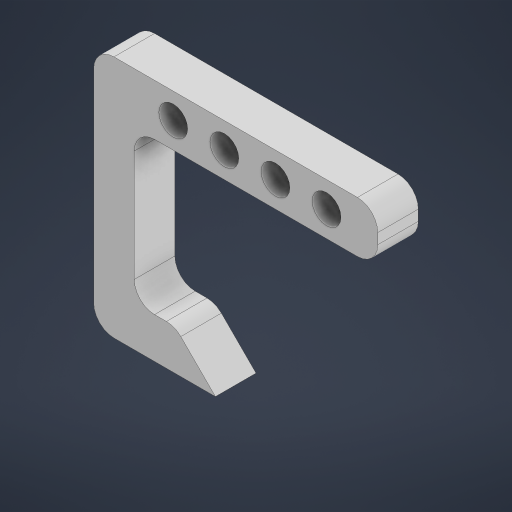
# Autodesk Inventor part: CS_Latch_Hooks
Saved by Autodesk Inventor 2023 (Build 270158000, 158)
## iProperties
Created: 2024-02-23
Part Number: CS_Latch_Hooks
Material: Generic
Document SubType Name: Modeling
Designer: kelle
Density: 1 g/cm^3
Appearance: Default
Author: kelle
Autodesk Inventor part; units mm, degrees
ref_plane "YZ Plane" through (0, 0, 0) normal (1, 0, 0) x (0, 1, 0)
ref_plane "XZ Plane" through (0, 0, 0) normal (0, 1, 0) x (-1, 0, 0)
ref_plane "XY Plane" through (0, 0, 0) normal (0, 0, 1) x (1, 0, 0)
sketch "Sketch1" plane through (0, 0, 0) normal (0, 0, 1) x (1, 0, 0)
  line L0 (19.05, -4) -> (-19.05, -4)
  line L1 (-19.05, -4) -> (-19.05, 4)
  line L2 (-19.05, 4) -> (19.05, 4)
  line L3 (19.05, 4) -> (19.05, -4)
  line L4 (19.05, -4) -> (-19.05, 4) construction
  line L5 (-19.05, -4) -> (19.05, 4) construction
  circle A0 centre (11.05, 0) radius 2.25
  circle A1 centre (3.05, 0) radius 2.25
  circle A2 centre (-4.95, 0) radius 2.25
  circle A3 centre (-12.95, 0) radius 2.25
  line L6 (-19.05, 4) -> (-25.4, 4)
  line L7 (-25.4, 4) -> (-25.4, -34.1)
  line L8 (-25.4, -34.1) -> (-19.05, -34.1)
  line L9 (-19.05, -34.1) -> (-19.05, 4)
  line L10 (-25.4, -34.1) -> (-12.6924, -34.1) construction
  line L11 (-25.4, -34.1) -> (-6.35, -34.1)
  line L12 (-6.35, -34.1) -> (-6.35, -27.75)
  line L13 (-6.35, -27.75) -> (-25.4, -27.75)
  line L14 (-25.4, -27.75) -> (-25.4, -34.1)
  line L15 (-6.35, -34.1) -> (-17.257, -23.193)
  point P0 (0, 0)
  point P1 (-19.05, -27.75)
  point P2 (-12.7, -27.75)
  point P3 (-19.05, -27.75)
  dimension "d0" = 38.1
  dimension "d1" = 8
  dimension "d2" = 4.5
  dimension "d3" = 8
  dimension "d4" = 4.5
  dimension "d5" = 8
  dimension "d6" = 4.5
  dimension "d7" = 8
  dimension "d8" = 4.5
  dimension "d9" = 8
  dimension "d10" = 4
  dimension "d11" = 4
  dimension "d12" = 4
  dimension "d13" = 4
  dimension "d16" = 6.35
  dimension "d17" = 38.1
  dimension "d20" = 19.05
  dimension "d21" = 6.35
  dimension "d22" = 45
  constraints: 32 end point, 6 parallel, 4 centre point, 4 horizontal, 3 perpendicular, 2 midpoint, 1 point on line
  measures "d0" distance of L1.end L2.end
  measures "d1" distance of L0.end L1.end
  measures "d2" diameter of A0
  measures "d3" distance from line of L3 A0.centre
  measures "d4" diameter of A1
  measures "d5" distance of A0.centre A1.centre
  measures "d6" diameter of A2
  measures "d7" distance of A1.centre A2.centre
  measures "d8" diameter of A3
  measures "d9" distance of A2.centre A3.centre
  measures "d10" distance from line of L0 A0.centre
  measures "d11" distance from line of L0 A1.centre
  measures "d12" distance from line of L0 A2.centre
  measures "d13" distance from line of L0 A3.centre
  measures "d16" distance of L8.end L7.end
  measures "d17" distance of L7.end L6.end
  measures "d20" distance of L13.end L12.end
  measures "d21" distance of L12.end L11.end
  measures "d22" angle of L11 L15
extrude "Extrusion1" add sketch "Sketch1" along normal blind 6.35 contours L0 L1 L2 L3 | L9 L13 L7 L6 L1 | L13 L15 L11 L9 | L9 L8 L7 L13
fillet "Fillet1" radius 3.175 5 edges at (-19.05, -27.75, 3.175) (-19.05, -4, 3.175) (-25.4, 4, 3.175) (19.05, 4, 3.175) (19.05, -4, 3.175)
fillet "Fillet2" radius 3.175 2 edges at (-12.7, -27.75, 3.175) (-25.4, -34.1, 3.175)
body "Solid1"
